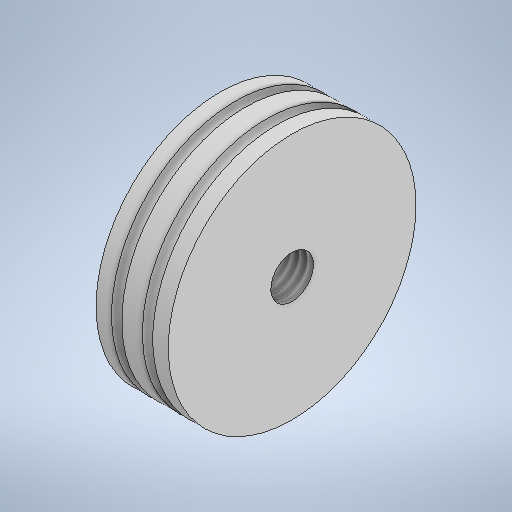
# Autodesk Inventor part: 40
Saved by Autodesk Inventor 2025.1 (Build 291241000, 241)
## iProperties
Created: 2024-09-17
Part Number: 40
Material: Generisch
Document SubType Name: Modeling
Designer: ffogue
Density: 1 g/cm^3
Appearance: Vorgabe
Author: ffogue
Autodesk Inventor part; units mm, degrees
ref_plane "YZ Plane" through (0, 0, 0) normal (1, 0, 0) x (0, 1, 0)
ref_plane "XZ Plane" through (0, 0, 0) normal (0, 1, 0) x (-1, 0, 0)
ref_plane "XY Plane" through (0, 0, 0) normal (0, 0, 1) x (1, 0, 0)
sketch "Sketch1" plane through (0, 0, 0) normal (0, 0, 1) x (1, 0, 0)
  line L0 (0, 0) -> (0, 12)
  line L1 (0, 12) -> (1.5, 12)
  line L2 (1.5, 12) -> (1.5, 12)
  line L3 (2.5, 12) -> (2.5, 12)
  line L4 (2.5, 12) -> (4.5, 12)
  line L5 (4.5, 12) -> (4.5, 12)
  line L6 (5.5, 12) -> (5.5, 12)
  line L7 (5.5, 12) -> (7, 12)
  line L8 (7, 12) -> (7, 0)
  line L9 (7, 0) -> (0, 0)
  arc A0 (1.5, 12) -> (2.5, 12) centre (2, 12) ccw
  arc A1 (4.5, 12) -> (5.5, 12) centre (5, 12) ccw
  point P0 (0.75, 12)
  dimension "d0" = 7
  dimension "d2" = 0.5
  dimension "d3" = 0.5
  dimension "d4" = 2
  dimension "d5" = 2
  dimension "d6" = 24
  constraints: 20 end point, 5 perpendicular, 4 point on circle, 4 point on line, 4 tangent, 2 centre point, 2 horizontal alignment, 1 coincident, 1 midpoint, 1 vertical
  measures "d0" distance of L8.end L0.start
  measures "d2" radius of A0
  measures "d3" radius of A1
  measures "d4" distance from line of L0 A0.centre
  measures "d5" distance from line of L8 A1.centre
  measures "d6" diameter of point (0.75, 12) L9
revolve "Revolution1" add sketch "Sketch1" angle 360 about axis through (7, 0, 0) along (-1, 0, 0)
sketch "Sketch2" plane through (0, 0, 0) normal (-1, 0, 0) x (0, 0, 1)
  circle A0 centre (0, 0) radius 12 projected
  point P0 (0, 0)
  constraints: 1 coincident
hole "Hole1" at (0, 0, 0) direction (1, 0, 0) diameter 10 depth 2
sketch "Sketch3" plane through (7, 0, 0) normal (1, 0, 0) x (0, 0, -1)
  circle A0 centre (0, 0) radius 12 projected
  constraints: 1 coincident
hole "Hole2" at (7, 0, 0) direction (-1, 0, 0) diameter 4.134 depth 5 thread size "M5x0.8" class "6H" standard "ISO Metric profile"
equation "\"d5\" = d4"
body "Solid1"
